Autodesk Fusion 360 part; units mm, degrees
note: some values were not read from the file. Set by a fixed rule: which sketch regions a step uses.
(part 2 of 2)
sketch "スケッチ7" plane through (0, 0, 8) normal (0, 0, 1) x (-1, 0, 0)
  arc A0 (19.6617, -4.7917) -> (19.8821, -5.409) centre (20.2564, -4.9274) ccw
  arc A1 (19.6617, -4.7917) -> (19.7936, -4.2138) centre (0, 0) ccw
  arc A2 (20.26, -3.7531) -> (19.7936, -4.2138) centre (20.3883, -4.3495) ccw
  line L0 (20.26, -3.7531) -> (20.9366, -3.6076)
  arc A3 (20.9366, -3.6076) -> (21.412, -3.0986) centre (20.8082, -3.0112) ccw
  arc A4 (21.412, -3.0986) -> (21.5646, -1.7437) centre (0, 0) ccw
  arc A5 (21.5646, -1.7437) -> (21.2144, -1.1417) centre (20.9566, -1.6945) ccw
  line L1 (21.2144, -1.1417) -> (20.5872, -0.8492)
  arc A6 (20.235, -0.2964) -> (20.5872, -0.8492) centre (20.845, -0.2964) ccw
  arc A7 (20.235, -0.2964) -> (20.235, 0.2964) centre (0, 0) ccw
  arc A8 (20.5872, 0.8492) -> (20.235, 0.2964) centre (20.845, 0.2964) ccw
  line L2 (20.5872, 0.8492) -> (21.2144, 1.1417)
  arc A9 (21.2144, 1.1417) -> (21.5646, 1.7437) centre (20.9566, 1.6945) ccw
  arc A10 (21.5646, 1.7437) -> (21.412, 3.0986) centre (0, 0) ccw
  arc A11 (21.412, 3.0986) -> (20.9366, 3.6076) centre (20.8082, 3.0112) ccw
  line L3 (20.9366, 3.6076) -> (20.26, 3.7531)
  arc A12 (19.7936, 4.2138) -> (20.26, 3.7531) centre (20.3883, 4.3495) ccw
  arc A13 (19.7936, 4.2138) -> (19.6617, 4.7917) centre (0, 0) ccw
  arc A14 (19.8821, 5.409) -> (19.6617, 4.7917) centre (20.2564, 4.9274) ccw
  line L4 (19.8821, 5.409) -> (20.4285, 5.8337)
  arc A15 (20.4285, 5.8337) -> (20.6359, 6.4986) centre (20.0541, 6.3153) ccw
  arc A16 (20.6359, 6.4986) -> (20.1856, 7.7855) centre (0, 0) ccw
  arc A17 (20.1856, 7.7855) -> (19.6089, 8.1759) centre (19.6165, 7.566) ccw
  line L5 (19.6089, 8.1759) -> (18.9169, 8.1673)
  arc A18 (18.3597, 8.5126) -> (18.9169, 8.1673) centre (18.9093, 8.7773) ccw
  arc A19 (18.3597, 8.5126) -> (18.1025, 9.0467) centre (0, 0) ccw
  arc A20 (18.18, 9.6976) -> (18.1025, 9.0467) centre (18.6521, 9.3113) ccw
  line L6 (18.18, 9.6976) -> (18.6181, 10.2332)
  arc A21 (18.6181, 10.2332) -> (18.6725, 10.9276) centre (18.146, 10.6195) ccw
  arc A22 (18.6725, 10.9276) -> (17.9471, 12.082) centre (0, 0) ccw
  arc A23 (17.9471, 12.082) -> (17.2979, 12.3343) centre (17.4411, 11.7414) ccw
  line L7 (17.2979, 12.3343) -> (16.6252, 12.172)
  arc A24 (16.0052, 12.3846) -> (16.6252, 12.172) centre (16.4821, 12.7649) ccw
  arc A25 (16.0052, 12.3846) -> (15.6356, 12.848) centre (0, 0) ccw
  arc A26 (15.5662, 13.4999) -> (15.6356, 12.848) centre (16.1125, 13.2284) ccw
  line L8 (15.5662, 13.4999) -> (15.8742, 14.1196)
  arc A27 (15.8742, 14.1196) -> (15.7727, 14.8086) centre (15.328, 14.3911) ccw
  arc A28 (15.7727, 14.8086) -> (14.8086, 15.7727) centre (0, 0) ccw
  arc A29 (14.8086, 15.7727) -> (14.1196, 15.8742) centre (14.3911, 15.328) ccw
  line L9 (14.1196, 15.8742) -> (13.4999, 15.5662)
  arc A30 (12.848, 15.6356) -> (13.4999, 15.5662) centre (13.2284, 16.1125) ccw
  arc A31 (12.848, 15.6356) -> (12.3846, 16.0052) centre (0, 0) ccw
  arc A32 (12.172, 16.6252) -> (12.3846, 16.0052) centre (12.7649, 16.4821) ccw
  line L10 (12.172, 16.6252) -> (12.3343, 17.2979)
  arc A33 (12.3343, 17.2979) -> (12.082, 17.9471) centre (11.7414, 17.4411) ccw
  arc A34 (12.082, 17.9471) -> (10.9276, 18.6725) centre (0, 0) ccw
  arc A35 (10.9276, 18.6725) -> (10.2332, 18.6181) centre (10.6195, 18.146) ccw
  line L11 (10.2332, 18.6181) -> (9.6976, 18.18)
  arc A36 (9.0467, 18.1025) -> (9.6976, 18.18) centre (9.3113, 18.6521) ccw
  arc A37 (9.0467, 18.1025) -> (8.5126, 18.3597) centre (0, 0) ccw
  arc A38 (8.1673, 18.9169) -> (8.5126, 18.3597) centre (8.7773, 18.9093) ccw
  line L12 (8.1673, 18.9169) -> (8.1759, 19.6089)
  arc A39 (8.1759, 19.6089) -> (7.7855, 20.1856) centre (7.566, 19.6165) ccw
  arc A40 (7.7855, 20.1856) -> (6.4986, 20.6359) centre (0, 0) ccw
  arc A41 (6.4986, 20.6359) -> (5.8337, 20.4285) centre (6.3153, 20.0541) ccw
  line L13 (5.8337, 20.4285) -> (5.409, 19.8821)
  arc A42 (4.7917, 19.6617) -> (5.409, 19.8821) centre (4.9274, 20.2564) ccw
  arc A43 (4.7917, 19.6617) -> (4.2138, 19.7936) centre (0, 0) ccw
  arc A44 (3.7531, 20.26) -> (4.2138, 19.7936) centre (4.3495, 20.3883) ccw
  line L14 (3.7531, 20.26) -> (3.6076, 20.9366)
  arc A45 (3.6076, 20.9366) -> (3.0986, 21.412) centre (3.0112, 20.8082) ccw
  arc A46 (3.0986, 21.412) -> (1.7437, 21.5646) centre (0, 0) ccw
  arc A47 (1.7437, 21.5646) -> (1.1417, 21.2144) centre (1.6945, 20.9566) ccw
  line L15 (1.1417, 21.2144) -> (0.8492, 20.5872)
  arc A48 (0.2964, 20.235) -> (0.8492, 20.5872) centre (0.2964, 20.845) ccw
  arc A49 (0.2964, 20.235) -> (-0.2964, 20.235) centre (0, 0) ccw
  arc A50 (-0.8492, 20.5872) -> (-0.2964, 20.235) centre (-0.2964, 20.845) ccw
  line L16 (-0.8492, 20.5872) -> (-1.1417, 21.2144)
  arc A51 (-1.1417, 21.2144) -> (-1.7437, 21.5646) centre (-1.6945, 20.9566) ccw
  arc A52 (-1.7437, 21.5646) -> (-3.0986, 21.412) centre (0, 0) ccw
  arc A53 (-3.0986, 21.412) -> (-3.6076, 20.9366) centre (-3.0112, 20.8082) ccw
  line L17 (-3.6076, 20.9366) -> (-3.7531, 20.26)
  arc A54 (-4.2138, 19.7936) -> (-3.7531, 20.26) centre (-4.3495, 20.3883) ccw
  arc A55 (-4.2138, 19.7936) -> (-4.7917, 19.6617) centre (0, 0) ccw
  arc A56 (-5.409, 19.8821) -> (-4.7917, 19.6617) centre (-4.9274, 20.2564) ccw
  line L18 (-5.409, 19.8821) -> (-5.8337, 20.4285)
  arc A57 (-5.8337, 20.4285) -> (-6.4986, 20.6359) centre (-6.3153, 20.0541) ccw
  arc A58 (-6.4986, 20.6359) -> (-7.7855, 20.1856) centre (0, 0) ccw
  arc A59 (-7.7855, 20.1856) -> (-8.1759, 19.6089) centre (-7.566, 19.6165) ccw
  line L19 (-8.1759, 19.6089) -> (-8.1673, 18.9169)
  arc A60 (-8.5126, 18.3597) -> (-8.1673, 18.9169) centre (-8.7773, 18.9093) ccw
  arc A61 (-8.5126, 18.3597) -> (-9.0467, 18.1025) centre (0, 0) ccw
  arc A62 (-9.6976, 18.18) -> (-9.0467, 18.1025) centre (-9.3113, 18.6521) ccw
  line L20 (-9.6976, 18.18) -> (-10.2332, 18.6181)
  arc A63 (-10.2332, 18.6181) -> (-10.9276, 18.6725) centre (-10.6195, 18.146) ccw
  arc A64 (-10.9276, 18.6725) -> (-12.082, 17.9471) centre (0, 0) ccw
  arc A65 (-12.082, 17.9471) -> (-12.3343, 17.2979) centre (-11.7414, 17.4411) ccw
  line L21 (-12.3343, 17.2979) -> (-12.172, 16.6252)
  arc A66 (-12.3846, 16.0052) -> (-12.172, 16.6252) centre (-12.7649, 16.4821) ccw
  arc A67 (-12.3846, 16.0052) -> (-12.848, 15.6356) centre (0, 0) ccw
  arc A68 (-13.4999, 15.5662) -> (-12.848, 15.6356) centre (-13.2284, 16.1125) ccw
  line L22 (-13.4999, 15.5662) -> (-14.1196, 15.8742)
  arc A69 (-14.1196, 15.8742) -> (-14.8086, 15.7727) centre (-14.3911, 15.328) ccw
  arc A70 (-14.8086, 15.7727) -> (-15.7727, 14.8086) centre (0, 0) ccw
  arc A71 (-15.7727, 14.8086) -> (-15.8742, 14.1196) centre (-15.328, 14.3911) ccw
  line L23 (-15.8742, 14.1196) -> (-15.5662, 13.4999)
  arc A72 (-15.6356, 12.848) -> (-15.5662, 13.4999) centre (-16.1125, 13.2284) ccw
  arc A73 (-15.6356, 12.848) -> (-16.0052, 12.3846) centre (0, 0) ccw
  arc A74 (-16.6252, 12.172) -> (-16.0052, 12.3846) centre (-16.4821, 12.7649) ccw
  line L24 (-16.6252, 12.172) -> (-17.2979, 12.3343)
  arc A75 (-17.2979, 12.3343) -> (-17.9471, 12.082) centre (-17.4411, 11.7414) ccw
  arc A76 (-17.9471, 12.082) -> (-18.6725, 10.9276) centre (0, 0) ccw
  arc A77 (-18.6725, 10.9276) -> (-18.6181, 10.2332) centre (-18.146, 10.6195) ccw
  line L25 (-18.6181, 10.2332) -> (-18.18, 9.6976)
  arc A78 (-18.1025, 9.0467) -> (-18.18, 9.6976) centre (-18.6521, 9.3113) ccw
  arc A79 (-18.1025, 9.0467) -> (-18.3597, 8.5126) centre (0, 0) ccw
  arc A80 (-18.9169, 8.1673) -> (-18.3597, 8.5126) centre (-18.9093, 8.7773) ccw
  line L26 (-18.9169, 8.1673) -> (-19.6089, 8.1759)
  arc A81 (-19.6089, 8.1759) -> (-20.1856, 7.7855) centre (-19.6165, 7.566) ccw
  arc A82 (-20.1856, 7.7855) -> (-20.6359, 6.4986) centre (0, 0) ccw
  arc A83 (-20.6359, 6.4986) -> (-20.4285, 5.8337) centre (-20.0541, 6.3153) ccw
  line L27 (-20.4285, 5.8337) -> (-19.8821, 5.409)
  arc A84 (-19.6617, 4.7917) -> (-19.8821, 5.409) centre (-20.2564, 4.9274) ccw
  arc A85 (-19.6617, 4.7917) -> (-19.7936, 4.2138) centre (0, 0) ccw
  arc A86 (-20.26, 3.7531) -> (-19.7936, 4.2138) centre (-20.3883, 4.3495) ccw
  line L28 (-20.26, 3.7531) -> (-20.9366, 3.6076)
  arc A87 (-20.9366, 3.6076) -> (-21.412, 3.0986) centre (-20.8082, 3.0112) ccw
  arc A88 (-21.412, 3.0986) -> (-21.5646, 1.7437) centre (0, 0) ccw
  arc A89 (-21.5646, 1.7437) -> (-21.2144, 1.1417) centre (-20.9566, 1.6945) ccw
  line L29 (-21.2144, 1.1417) -> (-20.5872, 0.8492)
  arc A90 (-20.235, 0.2964) -> (-20.5872, 0.8492) centre (-20.845, 0.2964) ccw
  arc A91 (-20.235, 0.2964) -> (-20.235, -0.2964) centre (0, 0) ccw
  arc A92 (-20.5872, -0.8492) -> (-20.235, -0.2964) centre (-20.845, -0.2964) ccw
  line L30 (-20.5872, -0.8492) -> (-21.2144, -1.1417)
  arc A93 (-21.2144, -1.1417) -> (-21.5646, -1.7437) centre (-20.9566, -1.6945) ccw
  arc A94 (-21.5646, -1.7437) -> (-21.412, -3.0986) centre (0, 0) ccw
  arc A95 (-21.412, -3.0986) -> (-20.9366, -3.6076) centre (-20.8082, -3.0112) ccw
  line L31 (-20.9366, -3.6076) -> (-20.26, -3.7531)
  arc A96 (-19.7936, -4.2138) -> (-20.26, -3.7531) centre (-20.3883, -4.3495) ccw
  arc A97 (-19.7936, -4.2138) -> (-19.6617, -4.7917) centre (0, 0) ccw
  arc A98 (-19.8821, -5.409) -> (-19.6617, -4.7917) centre (-20.2564, -4.9274) ccw
  line L32 (-19.8821, -5.409) -> (-20.4285, -5.8337)
  arc A99 (-20.4285, -5.8337) -> (-20.6359, -6.4986) centre (-20.0541, -6.3153) ccw
  arc A100 (-20.6359, -6.4986) -> (-20.1856, -7.7855) centre (0, 0) ccw
  arc A101 (-20.1856, -7.7855) -> (-19.6089, -8.1759) centre (-19.6165, -7.566) ccw
  line L33 (-19.6089, -8.1759) -> (-18.9169, -8.1673)
  arc A102 (-18.3597, -8.5126) -> (-18.9169, -8.1673) centre (-18.9093, -8.7773) ccw
  arc A103 (-18.3597, -8.5126) -> (-18.1025, -9.0467) centre (0, 0) ccw
  arc A104 (-18.18, -9.6976) -> (-18.1025, -9.0467) centre (-18.6521, -9.3113) ccw
  line L34 (-18.18, -9.6976) -> (-18.6181, -10.2332)
  arc A105 (-18.6181, -10.2332) -> (-18.6725, -10.9276) centre (-18.146, -10.6195) ccw
  arc A106 (-18.6725, -10.9276) -> (-17.9471, -12.082) centre (0, 0) ccw
  arc A107 (-17.9471, -12.082) -> (-17.2979, -12.3343) centre (-17.4411, -11.7414) ccw
  line L35 (-17.2979, -12.3343) -> (-16.6252, -12.172)
  arc A108 (-16.0052, -12.3846) -> (-16.6252, -12.172) centre (-16.4821, -12.7649) ccw
  arc A109 (-16.0052, -12.3846) -> (-15.6356, -12.848) centre (0, 0) ccw
  arc A110 (-15.5662, -13.4999) -> (-15.6356, -12.848) centre (-16.1125, -13.2284) ccw
  line L36 (-15.5662, -13.4999) -> (-15.8742, -14.1196)
  arc A111 (-15.8742, -14.1196) -> (-15.7727, -14.8086) centre (-15.328, -14.3911) ccw
  arc A112 (-15.7727, -14.8086) -> (-14.8086, -15.7727) centre (0, 0) ccw
  arc A113 (-14.8086, -15.7727) -> (-14.1196, -15.8742) centre (-14.3911, -15.328) ccw
  line L37 (-14.1196, -15.8742) -> (-13.4999, -15.5662)
  arc A114 (-12.848, -15.6356) -> (-13.4999, -15.5662) centre (-13.2284, -16.1125) ccw
  arc A115 (-12.848, -15.6356) -> (-12.3846, -16.0052) centre (0, 0) ccw
  arc A116 (-12.172, -16.6252) -> (-12.3846, -16.0052) centre (-12.7649, -16.4821) ccw
  line L38 (-12.172, -16.6252) -> (-12.3343, -17.2979)
  arc A117 (-12.3343, -17.2979) -> (-12.082, -17.9471) centre (-11.7414, -17.4411) ccw
  arc A118 (-12.082, -17.9471) -> (-10.9276, -18.6725) centre (0, 0) ccw
  arc A119 (-10.9276, -18.6725) -> (-10.2332, -18.6181) centre (-10.6195, -18.146) ccw
  line L39 (-10.2332, -18.6181) -> (-9.6976, -18.18)
  arc A120 (-9.0467, -18.1025) -> (-9.6976, -18.18) centre (-9.3113, -18.6521) ccw
  arc A121 (-9.0467, -18.1025) -> (-8.5126, -18.3597) centre (0, 0) ccw
  arc A122 (-8.1673, -18.9169) -> (-8.5126, -18.3597) centre (-8.7773, -18.9093) ccw
  line L40 (-8.1673, -18.9169) -> (-8.1759, -19.6089)
  arc A123 (-8.1759, -19.6089) -> (-7.7855, -20.1856) centre (-7.566, -19.6165) ccw
  arc A124 (-7.7855, -20.1856) -> (-6.4986, -20.6359) centre (0, 0) ccw
  arc A125 (-6.4986, -20.6359) -> (-5.8337, -20.4285) centre (-6.3153, -20.0541) ccw
  line L41 (-5.8337, -20.4285) -> (-5.409, -19.8821)
  arc A126 (-4.7917, -19.6617) -> (-5.409, -19.8821) centre (-4.9274, -20.2564) ccw
  arc A127 (-4.7917, -19.6617) -> (-4.2138, -19.7936) centre (0, 0) ccw
  arc A128 (-3.7531, -20.26) -> (-4.2138, -19.7936) centre (-4.3495, -20.3883) ccw
  line L42 (-3.7531, -20.26) -> (-3.6076, -20.9366)
  arc A129 (-3.6076, -20.9366) -> (-3.0986, -21.412) centre (-3.0112, -20.8082) ccw
  arc A130 (-3.0986, -21.412) -> (-1.7437, -21.5646) centre (0, 0) ccw
  arc A131 (-1.7437, -21.5646) -> (-1.1417, -21.2144) centre (-1.6945, -20.9566) ccw
  line L43 (-1.1417, -21.2144) -> (-0.8492, -20.5872)
  arc A132 (-0.2964, -20.235) -> (-0.8492, -20.5872) centre (-0.2964, -20.845) ccw
  arc A133 (-0.2964, -20.235) -> (0.2964, -20.235) centre (0, 0) ccw
  arc A134 (0.8492, -20.5872) -> (0.2964, -20.235) centre (0.2964, -20.845) ccw
  line L44 (0.8492, -20.5872) -> (1.1417, -21.2144)
  arc A135 (1.1417, -21.2144) -> (1.7437, -21.5646) centre (1.6945, -20.9566) ccw
  arc A136 (1.7437, -21.5646) -> (3.0986, -21.412) centre (0, 0) ccw
  arc A137 (3.0986, -21.412) -> (3.6076, -20.9366) centre (3.0112, -20.8082) ccw
  line L45 (3.6076, -20.9366) -> (3.7531, -20.26)
  arc A138 (4.2138, -19.7936) -> (3.7531, -20.26) centre (4.3495, -20.3883) ccw
  arc A139 (4.2138, -19.7936) -> (4.7917, -19.6617) centre (0, 0) ccw
  arc A140 (5.409, -19.8821) -> (4.7917, -19.6617) centre (4.9274, -20.2564) ccw
  line L46 (5.409, -19.8821) -> (5.8337, -20.4285)
  arc A141 (5.8337, -20.4285) -> (6.4986, -20.6359) centre (6.3153, -20.0541) ccw
  arc A142 (6.4986, -20.6359) -> (7.7855, -20.1856) centre (0, 0) ccw
  arc A143 (7.7855, -20.1856) -> (8.1759, -19.6089) centre (7.566, -19.6165) ccw
  line L47 (8.1759, -19.6089) -> (8.1673, -18.9169)
  arc A144 (8.5126, -18.3597) -> (8.1673, -18.9169) centre (8.7773, -18.9093) ccw
  arc A145 (8.5126, -18.3597) -> (9.0467, -18.1025) centre (0, 0) ccw
  arc A146 (9.6976, -18.18) -> (9.0467, -18.1025) centre (9.3113, -18.6521) ccw
  line L48 (9.6976, -18.18) -> (10.2332, -18.6181)
  arc A147 (10.2332, -18.6181) -> (10.9276, -18.6725) centre (10.6195, -18.146) ccw
  arc A148 (10.9276, -18.6725) -> (12.082, -17.9471) centre (0, 0) ccw
  arc A149 (12.082, -17.9471) -> (12.3343, -17.2979) centre (11.7414, -17.4411) ccw
  line L49 (12.3343, -17.2979) -> (12.172, -16.6252)
  arc A150 (12.3846, -16.0052) -> (12.172, -16.6252) centre (12.7649, -16.4821) ccw
  arc A151 (12.3846, -16.0052) -> (12.848, -15.6356) centre (0, 0) ccw
  arc A152 (13.4999, -15.5662) -> (12.848, -15.6356) centre (13.2284, -16.1125) ccw
  line L50 (13.4999, -15.5662) -> (14.1196, -15.8742)
  arc A153 (14.1196, -15.8742) -> (14.8086, -15.7727) centre (14.3911, -15.328) ccw
  arc A154 (14.8086, -15.7727) -> (15.7727, -14.8086) centre (0, 0) ccw
  arc A155 (15.7727, -14.8086) -> (15.8742, -14.1196) centre (15.328, -14.3911) ccw
  line L51 (15.8742, -14.1196) -> (15.5662, -13.4999)
  arc A156 (15.6356, -12.848) -> (15.5662, -13.4999) centre (16.1125, -13.2284) ccw
  arc A157 (15.6356, -12.848) -> (16.0052, -12.3846) centre (0, 0) ccw
  arc A158 (16.6252, -12.172) -> (16.0052, -12.3846) centre (16.4821, -12.7649) ccw
  line L52 (16.6252, -12.172) -> (17.2979, -12.3343)
  arc A159 (17.2979, -12.3343) -> (17.9471, -12.082) centre (17.4411, -11.7414) ccw
  arc A160 (17.9471, -12.082) -> (18.6725, -10.9276) centre (0, 0) ccw
  arc A161 (18.6725, -10.9276) -> (18.6181, -10.2332) centre (18.146, -10.6195) ccw
  line L53 (18.6181, -10.2332) -> (18.18, -9.6976)
  arc A162 (18.1025, -9.0467) -> (18.18, -9.6976) centre (18.6521, -9.3113) ccw
  arc A163 (18.1025, -9.0467) -> (18.3597, -8.5126) centre (0, 0) ccw
  arc A164 (18.9169, -8.1673) -> (18.3597, -8.5126) centre (18.9093, -8.7773) ccw
  line L54 (18.9169, -8.1673) -> (19.6089, -8.1759)
  arc A165 (19.6089, -8.1759) -> (20.1856, -7.7855) centre (19.6165, -7.566) ccw
  arc A166 (20.1856, -7.7855) -> (20.6359, -6.4986) centre (0, 0) ccw
  arc A167 (20.6359, -6.4986) -> (20.4285, -5.8337) centre (20.0541, -6.3153) ccw
  line L55 (20.4285, -5.8337) -> (19.8821, -5.409)
  line L56 (-0.3, 3) -> (0.3, 3)
  line L57 (0.3, 3) -> (0.3, -3)
  line L58 (0.3, -3) -> (-0.3, -3)
  line L59 (-0.3, -3) -> (-0.3, 3)
  line L60 (-0.3, 3) -> (0.3, -3) construction
  line L61 (0.3, 3) -> (-0.3, -3) construction
  circle A168 centre (-0.3, 0) radius 3
  circle A169 centre (0.3, 0) radius 3
  dimension "d78" = 0.6
  dimension "d79" = 6
  constraint horizontal L56
  constraint perpendicular L56 L57
  constraint parallel L56 L58
  constraint parallel L57 L59
  constraint coincident L60 A1.centre
  constraint coincident L61 A1.centre
  constraint coincident A1.centre A4.centre
  constraint midpoint L59 A168.centre
  constraint coincident L58.end A168
  constraint midpoint L57 A169.centre
  constraint coincident L57.end A169
  measures "d78" distance of L57.end L58.end
  measures "d79" distance of L56.end L57.end
extrude "押し出し7" cut sketch "スケッチ7" against normal blind 8 contours L59 A168 A169 | L57 A168 A169 | L59 A169 | L57 A168 picked at (-2.9825, -0.8024) picked at (3.04, 0.5606)
cylinder "円柱プリミティブ1" cut diameter 8 height -8 placed x (1, 0, 0) y (0, 1, 0) z (0, 0, 1) at (0, 0, 8)
sketch "スケッチ9" plane through (0, 0, 8) normal (0, 0, 1) x (-1, 0, 0)
  circle A0 centre (0, 0) radius 4
  arc A1 (19.6617, -4.7917) -> (19.8821, -5.409) centre (20.2564, -4.9274) ccw
  arc A2 (19.6617, -4.7917) -> (19.7936, -4.2138) centre (0, 0) ccw
  arc A3 (20.26, -3.7531) -> (19.7936, -4.2138) centre (20.3883, -4.3495) ccw
  line L0 (20.26, -3.7531) -> (20.9366, -3.6076)
  arc A4 (20.9366, -3.6076) -> (21.412, -3.0986) centre (20.8082, -3.0112) ccw
  arc A5 (21.412, -3.0986) -> (21.5646, -1.7437) centre (0, 0) ccw
  arc A6 (21.5646, -1.7437) -> (21.2144, -1.1417) centre (20.9566, -1.6945) ccw
  line L1 (21.2144, -1.1417) -> (20.5872, -0.8492)
  arc A7 (20.235, -0.2964) -> (20.5872, -0.8492) centre (20.845, -0.2964) ccw
  arc A8 (20.235, -0.2964) -> (20.235, 0.2964) centre (0, 0) ccw
  arc A9 (20.5872, 0.8492) -> (20.235, 0.2964) centre (20.845, 0.2964) ccw
  line L2 (20.5872, 0.8492) -> (21.2144, 1.1417)
  arc A10 (21.2144, 1.1417) -> (21.5646, 1.7437) centre (20.9566, 1.6945) ccw
  arc A11 (21.5646, 1.7437) -> (21.412, 3.0986) centre (0, 0) ccw
  arc A12 (21.412, 3.0986) -> (20.9366, 3.6076) centre (20.8082, 3.0112) ccw
  line L3 (20.9366, 3.6076) -> (20.26, 3.7531)
  arc A13 (19.7936, 4.2138) -> (20.26, 3.7531) centre (20.3883, 4.3495) ccw
  arc A14 (19.7936, 4.2138) -> (19.6617, 4.7917) centre (0, 0) ccw
  arc A15 (19.8821, 5.409) -> (19.6617, 4.7917) centre (20.2564, 4.9274) ccw
  line L4 (19.8821, 5.409) -> (20.4285, 5.8337)
  arc A16 (20.4285, 5.8337) -> (20.6359, 6.4986) centre (20.0541, 6.3153) ccw
  arc A17 (20.6359, 6.4986) -> (20.1856, 7.7855) centre (0, 0) ccw
  arc A18 (20.1856, 7.7855) -> (19.6089, 8.1759) centre (19.6165, 7.566) ccw
  line L5 (19.6089, 8.1759) -> (18.9169, 8.1673)
  arc A19 (18.3597, 8.5126) -> (18.9169, 8.1673) centre (18.9093, 8.7773) ccw
  arc A20 (18.3597, 8.5126) -> (18.1025, 9.0467) centre (0, 0) ccw
  arc A21 (18.18, 9.6976) -> (18.1025, 9.0467) centre (18.6521, 9.3113) ccw
  line L6 (18.18, 9.6976) -> (18.6181, 10.2332)
  arc A22 (18.6181, 10.2332) -> (18.6725, 10.9276) centre (18.146, 10.6195) ccw
  arc A23 (18.6725, 10.9276) -> (17.9471, 12.082) centre (0, 0) ccw
  arc A24 (17.9471, 12.082) -> (17.2979, 12.3343) centre (17.4411, 11.7414) ccw
  line L7 (17.2979, 12.3343) -> (16.6252, 12.172)
  arc A25 (16.0052, 12.3846) -> (16.6252, 12.172) centre (16.4821, 12.7649) ccw
  arc A26 (16.0052, 12.3846) -> (15.6356, 12.848) centre (0, 0) ccw
  arc A27 (15.5662, 13.4999) -> (15.6356, 12.848) centre (16.1125, 13.2284) ccw
  line L8 (15.5662, 13.4999) -> (15.8742, 14.1196)
  arc A28 (15.8742, 14.1196) -> (15.7727, 14.8086) centre (15.328, 14.3911) ccw
  arc A29 (15.7727, 14.8086) -> (14.8086, 15.7727) centre (0, 0) ccw
  arc A30 (14.8086, 15.7727) -> (14.1196, 15.8742) centre (14.3911, 15.328) ccw
  line L9 (14.1196, 15.8742) -> (13.4999, 15.5662)
  arc A31 (12.848, 15.6356) -> (13.4999, 15.5662) centre (13.2284, 16.1125) ccw
  arc A32 (12.848, 15.6356) -> (12.3846, 16.0052) centre (0, 0) ccw
  arc A33 (12.172, 16.6252) -> (12.3846, 16.0052) centre (12.7649, 16.4821) ccw
  line L10 (12.172, 16.6252) -> (12.3343, 17.2979)
  arc A34 (12.3343, 17.2979) -> (12.082, 17.9471) centre (11.7414, 17.4411) ccw
  arc A35 (12.082, 17.9471) -> (10.9276, 18.6725) centre (0, 0) ccw
  arc A36 (10.9276, 18.6725) -> (10.2332, 18.6181) centre (10.6195, 18.146) ccw
  line L11 (10.2332, 18.6181) -> (9.6976, 18.18)
  arc A37 (9.0467, 18.1025) -> (9.6976, 18.18) centre (9.3113, 18.6521) ccw
  arc A38 (9.0467, 18.1025) -> (8.5126, 18.3597) centre (0, 0) ccw
  arc A39 (8.1673, 18.9169) -> (8.5126, 18.3597) centre (8.7773, 18.9093) ccw
  line L12 (8.1673, 18.9169) -> (8.1759, 19.6089)
  arc A40 (8.1759, 19.6089) -> (7.7855, 20.1856) centre (7.566, 19.6165) ccw
  arc A41 (7.7855, 20.1856) -> (6.4986, 20.6359) centre (0, 0) ccw
  arc A42 (6.4986, 20.6359) -> (5.8337, 20.4285) centre (6.3153, 20.0541) ccw
  line L13 (5.8337, 20.4285) -> (5.409, 19.8821)
  arc A43 (4.7917, 19.6617) -> (5.409, 19.8821) centre (4.9274, 20.2564) ccw
  arc A44 (4.7917, 19.6617) -> (4.2138, 19.7936) centre (0, 0) ccw
  arc A45 (3.7531, 20.26) -> (4.2138, 19.7936) centre (4.3495, 20.3883) ccw
  line L14 (3.7531, 20.26) -> (3.6076, 20.9366)
  arc A46 (3.6076, 20.9366) -> (3.0986, 21.412) centre (3.0112, 20.8082) ccw
  arc A47 (3.0986, 21.412) -> (1.7437, 21.5646) centre (0, 0) ccw
  arc A48 (1.7437, 21.5646) -> (1.1417, 21.2144) centre (1.6945, 20.9566) ccw
  line L15 (1.1417, 21.2144) -> (0.8492, 20.5872)
  arc A49 (0.2964, 20.235) -> (0.8492, 20.5872) centre (0.2964, 20.845) ccw
  arc A50 (0.2964, 20.235) -> (-0.2964, 20.235) centre (0, 0) ccw
  arc A51 (-0.8492, 20.5872) -> (-0.2964, 20.235) centre (-0.2964, 20.845) ccw
  line L16 (-0.8492, 20.5872) -> (-1.1417, 21.2144)
  arc A52 (-1.1417, 21.2144) -> (-1.7437, 21.5646) centre (-1.6945, 20.9566) ccw
  arc A53 (-1.7437, 21.5646) -> (-3.0986, 21.412) centre (0, 0) ccw
  arc A54 (-3.0986, 21.412) -> (-3.6076, 20.9366) centre (-3.0112, 20.8082) ccw
  line L17 (-3.6076, 20.9366) -> (-3.7531, 20.26)
  arc A55 (-4.2138, 19.7936) -> (-3.7531, 20.26) centre (-4.3495, 20.3883) ccw
  arc A56 (-4.2138, 19.7936) -> (-4.7917, 19.6617) centre (0, 0) ccw
  arc A57 (-5.409, 19.8821) -> (-4.7917, 19.6617) centre (-4.9274, 20.2564) ccw
  line L18 (-5.409, 19.8821) -> (-5.8337, 20.4285)
  arc A58 (-5.8337, 20.4285) -> (-6.4986, 20.6359) centre (-6.3153, 20.0541) ccw
  arc A59 (-6.4986, 20.6359) -> (-7.7855, 20.1856) centre (0, 0) ccw
  arc A60 (-7.7855, 20.1856) -> (-8.1759, 19.6089) centre (-7.566, 19.6165) ccw
  line L19 (-8.1759, 19.6089) -> (-8.1673, 18.9169)
  arc A61 (-8.5126, 18.3597) -> (-8.1673, 18.9169) centre (-8.7773, 18.9093) ccw
  arc A62 (-8.5126, 18.3597) -> (-9.0467, 18.1025) centre (0, 0) ccw
  arc A63 (-9.6976, 18.18) -> (-9.0467, 18.1025) centre (-9.3113, 18.6521) ccw
  line L20 (-9.6976, 18.18) -> (-10.2332, 18.6181)
  arc A64 (-10.2332, 18.6181) -> (-10.9276, 18.6725) centre (-10.6195, 18.146) ccw
  arc A65 (-10.9276, 18.6725) -> (-12.082, 17.9471) centre (0, 0) ccw
  arc A66 (-12.082, 17.9471) -> (-12.3343, 17.2979) centre (-11.7414, 17.4411) ccw
  line L21 (-12.3343, 17.2979) -> (-12.172, 16.6252)
  arc A67 (-12.3846, 16.0052) -> (-12.172, 16.6252) centre (-12.7649, 16.4821) ccw
  arc A68 (-12.3846, 16.0052) -> (-12.848, 15.6356) centre (0, 0) ccw
  arc A69 (-13.4999, 15.5662) -> (-12.848, 15.6356) centre (-13.2284, 16.1125) ccw
  line L22 (-13.4999, 15.5662) -> (-14.1196, 15.8742)
  arc A70 (-14.1196, 15.8742) -> (-14.8086, 15.7727) centre (-14.3911, 15.328) ccw
  arc A71 (-14.8086, 15.7727) -> (-15.7727, 14.8086) centre (0, 0) ccw
  arc A72 (-15.7727, 14.8086) -> (-15.8742, 14.1196) centre (-15.328, 14.3911) ccw
  line L23 (-15.8742, 14.1196) -> (-15.5662, 13.4999)
  arc A73 (-15.6356, 12.848) -> (-15.5662, 13.4999) centre (-16.1125, 13.2284) ccw
  arc A74 (-15.6356, 12.848) -> (-16.0052, 12.3846) centre (0, 0) ccw
  arc A75 (-16.6252, 12.172) -> (-16.0052, 12.3846) centre (-16.4821, 12.7649) ccw
  line L24 (-16.6252, 12.172) -> (-17.2979, 12.3343)
  arc A76 (-17.2979, 12.3343) -> (-17.9471, 12.082) centre (-17.4411, 11.7414) ccw
  arc A77 (-17.9471, 12.082) -> (-18.6725, 10.9276) centre (0, 0) ccw
  arc A78 (-18.6725, 10.9276) -> (-18.6181, 10.2332) centre (-18.146, 10.6195) ccw
  line L25 (-18.6181, 10.2332) -> (-18.18, 9.6976)
  arc A79 (-18.1025, 9.0467) -> (-18.18, 9.6976) centre (-18.6521, 9.3113) ccw
  arc A80 (-18.1025, 9.0467) -> (-18.3597, 8.5126) centre (0, 0) ccw
  arc A81 (-18.9169, 8.1673) -> (-18.3597, 8.5126) centre (-18.9093, 8.7773) ccw
  line L26 (-18.9169, 8.1673) -> (-19.6089, 8.1759)
  arc A82 (-19.6089, 8.1759) -> (-20.1856, 7.7855) centre (-19.6165, 7.566) ccw
  arc A83 (-20.1856, 7.7855) -> (-20.6359, 6.4986) centre (0, 0) ccw
  arc A84 (-20.6359, 6.4986) -> (-20.4285, 5.8337) centre (-20.0541, 6.3153) ccw
  line L27 (-20.4285, 5.8337) -> (-19.8821, 5.409)
  arc A85 (-19.6617, 4.7917) -> (-19.8821, 5.409) centre (-20.2564, 4.9274) ccw
  arc A86 (-19.6617, 4.7917) -> (-19.7936, 4.2138) centre (0, 0) ccw
  arc A87 (-20.26, 3.7531) -> (-19.7936, 4.2138) centre (-20.3883, 4.3495) ccw
  line L28 (-20.26, 3.7531) -> (-20.9366, 3.6076)
  arc A88 (-20.9366, 3.6076) -> (-21.412, 3.0986) centre (-20.8082, 3.0112) ccw
  arc A89 (-21.412, 3.0986) -> (-21.5646, 1.7437) centre (0, 0) ccw
  arc A90 (-21.5646, 1.7437) -> (-21.2144, 1.1417) centre (-20.9566, 1.6945) ccw
  line L29 (-21.2144, 1.1417) -> (-20.5872, 0.8492)
  arc A91 (-20.235, 0.2964) -> (-20.5872, 0.8492) centre (-20.845, 0.2964) ccw
  arc A92 (-20.235, 0.2964) -> (-20.235, -0.2964) centre (0, 0) ccw
  arc A93 (-20.5872, -0.8492) -> (-20.235, -0.2964) centre (-20.845, -0.2964) ccw
  line L30 (-20.5872, -0.8492) -> (-21.2144, -1.1417)
  arc A94 (-21.2144, -1.1417) -> (-21.5646, -1.7437) centre (-20.9566, -1.6945) ccw
  arc A95 (-21.5646, -1.7437) -> (-21.412, -3.0986) centre (0, 0) ccw
  arc A96 (-21.412, -3.0986) -> (-20.9366, -3.6076) centre (-20.8082, -3.0112) ccw
  line L31 (-20.9366, -3.6076) -> (-20.26, -3.7531)
  arc A97 (-19.7936, -4.2138) -> (-20.26, -3.7531) centre (-20.3883, -4.3495) ccw
  arc A98 (-19.7936, -4.2138) -> (-19.6617, -4.7917) centre (0, 0) ccw
  arc A99 (-19.8821, -5.409) -> (-19.6617, -4.7917) centre (-20.2564, -4.9274) ccw
  line L32 (-19.8821, -5.409) -> (-20.4285, -5.8337)
  arc A100 (-20.4285, -5.8337) -> (-20.6359, -6.4986) centre (-20.0541, -6.3153) ccw
  arc A101 (-20.6359, -6.4986) -> (-20.1856, -7.7855) centre (0, 0) ccw
  arc A102 (-20.1856, -7.7855) -> (-19.6089, -8.1759) centre (-19.6165, -7.566) ccw
  line L33 (-19.6089, -8.1759) -> (-18.9169, -8.1673)
  arc A103 (-18.3597, -8.5126) -> (-18.9169, -8.1673) centre (-18.9093, -8.7773) ccw
  arc A104 (-18.3597, -8.5126) -> (-18.1025, -9.0467) centre (0, 0) ccw
  arc A105 (-18.18, -9.6976) -> (-18.1025, -9.0467) centre (-18.6521, -9.3113) ccw
  line L34 (-18.18, -9.6976) -> (-18.6181, -10.2332)
  arc A106 (-18.6181, -10.2332) -> (-18.6725, -10.9276) centre (-18.146, -10.6195) ccw
  arc A107 (-18.6725, -10.9276) -> (-17.9471, -12.082) centre (0, 0) ccw
  arc A108 (-17.9471, -12.082) -> (-17.2979, -12.3343) centre (-17.4411, -11.7414) ccw
  line L35 (-17.2979, -12.3343) -> (-16.6252, -12.172)
  arc A109 (-16.0052, -12.3846) -> (-16.6252, -12.172) centre (-16.4821, -12.7649) ccw
  arc A110 (-16.0052, -12.3846) -> (-15.6356, -12.848) centre (0, 0) ccw
  arc A111 (-15.5662, -13.4999) -> (-15.6356, -12.848) centre (-16.1125, -13.2284) ccw
  line L36 (-15.5662, -13.4999) -> (-15.8742, -14.1196)
  arc A112 (-15.8742, -14.1196) -> (-15.7727, -14.8086) centre (-15.328, -14.3911) ccw
  arc A113 (-15.7727, -14.8086) -> (-14.8086, -15.7727) centre (0, 0) ccw
  arc A114 (-14.8086, -15.7727) -> (-14.1196, -15.8742) centre (-14.3911, -15.328) ccw
  line L37 (-14.1196, -15.8742) -> (-13.4999, -15.5662)
  arc A115 (-12.848, -15.6356) -> (-13.4999, -15.5662) centre (-13.2284, -16.1125) ccw
  arc A116 (-12.848, -15.6356) -> (-12.3846, -16.0052) centre (0, 0) ccw
  arc A117 (-12.172, -16.6252) -> (-12.3846, -16.0052) centre (-12.7649, -16.4821) ccw
  line L38 (-12.172, -16.6252) -> (-12.3343, -17.2979)
  arc A118 (-12.3343, -17.2979) -> (-12.082, -17.9471) centre (-11.7414, -17.4411) ccw
  arc A119 (-12.082, -17.9471) -> (-10.9276, -18.6725) centre (0, 0) ccw
  arc A120 (-10.9276, -18.6725) -> (-10.2332, -18.6181) centre (-10.6195, -18.146) ccw
  line L39 (-10.2332, -18.6181) -> (-9.6976, -18.18)
  arc A121 (-9.0467, -18.1025) -> (-9.6976, -18.18) centre (-9.3113, -18.6521) ccw
  arc A122 (-9.0467, -18.1025) -> (-8.5126, -18.3597) centre (0, 0) ccw
  arc A123 (-8.1673, -18.9169) -> (-8.5126, -18.3597) centre (-8.7773, -18.9093) ccw
  line L40 (-8.1673, -18.9169) -> (-8.1759, -19.6089)
  arc A124 (-8.1759, -19.6089) -> (-7.7855, -20.1856) centre (-7.566, -19.6165) ccw
  arc A125 (-7.7855, -20.1856) -> (-6.4986, -20.6359) centre (0, 0) ccw
  arc A126 (-6.4986, -20.6359) -> (-5.8337, -20.4285) centre (-6.3153, -20.0541) ccw
  line L41 (-5.8337, -20.4285) -> (-5.409, -19.8821)
  arc A127 (-4.7917, -19.6617) -> (-5.409, -19.8821) centre (-4.9274, -20.2564) ccw
  arc A128 (-4.7917, -19.6617) -> (-4.2138, -19.7936) centre (0, 0) ccw
  arc A129 (-3.7531, -20.26) -> (-4.2138, -19.7936) centre (-4.3495, -20.3883) ccw
  line L42 (-3.7531, -20.26) -> (-3.6076, -20.9366)
  arc A130 (-3.6076, -20.9366) -> (-3.0986, -21.412) centre (-3.0112, -20.8082) ccw
  arc A131 (-3.0986, -21.412) -> (-1.7437, -21.5646) centre (0, 0) ccw
  arc A132 (-1.7437, -21.5646) -> (-1.1417, -21.2144) centre (-1.6945, -20.9566) ccw
  line L43 (-1.1417, -21.2144) -> (-0.8492, -20.5872)
  arc A133 (-0.2964, -20.235) -> (-0.8492, -20.5872) centre (-0.2964, -20.845) ccw
  arc A134 (-0.2964, -20.235) -> (0.2964, -20.235) centre (0, 0) ccw
  arc A135 (0.8492, -20.5872) -> (0.2964, -20.235) centre (0.2964, -20.845) ccw
  line L44 (0.8492, -20.5872) -> (1.1417, -21.2144)
  arc A136 (1.1417, -21.2144) -> (1.7437, -21.5646) centre (1.6945, -20.9566) ccw
  arc A137 (1.7437, -21.5646) -> (3.0986, -21.412) centre (0, 0) ccw
  arc A138 (3.0986, -21.412) -> (3.6076, -20.9366) centre (3.0112, -20.8082) ccw
  line L45 (3.6076, -20.9366) -> (3.7531, -20.26)
  arc A139 (4.2138, -19.7936) -> (3.7531, -20.26) centre (4.3495, -20.3883) ccw
  arc A140 (4.2138, -19.7936) -> (4.7917, -19.6617) centre (0, 0) ccw
  arc A141 (5.409, -19.8821) -> (4.7917, -19.6617) centre (4.9274, -20.2564) ccw
  line L46 (5.409, -19.8821) -> (5.8337, -20.4285)
  arc A142 (5.8337, -20.4285) -> (6.4986, -20.6359) centre (6.3153, -20.0541) ccw
  arc A143 (6.4986, -20.6359) -> (7.7855, -20.1856) centre (0, 0) ccw
  arc A144 (7.7855, -20.1856) -> (8.1759, -19.6089) centre (7.566, -19.6165) ccw
  line L47 (8.1759, -19.6089) -> (8.1673, -18.9169)
  arc A145 (8.5126, -18.3597) -> (8.1673, -18.9169) centre (8.7773, -18.9093) ccw
  arc A146 (8.5126, -18.3597) -> (9.0467, -18.1025) centre (0, 0) ccw
  arc A147 (9.6976, -18.18) -> (9.0467, -18.1025) centre (9.3113, -18.6521) ccw
  line L48 (9.6976, -18.18) -> (10.2332, -18.6181)
  arc A148 (10.2332, -18.6181) -> (10.9276, -18.6725) centre (10.6195, -18.146) ccw
  arc A149 (10.9276, -18.6725) -> (12.082, -17.9471) centre (0, 0) ccw
  arc A150 (12.082, -17.9471) -> (12.3343, -17.2979) centre (11.7414, -17.4411) ccw
  line L49 (12.3343, -17.2979) -> (12.172, -16.6252)
  arc A151 (12.3846, -16.0052) -> (12.172, -16.6252) centre (12.7649, -16.4821) ccw
  arc A152 (12.3846, -16.0052) -> (12.848, -15.6356) centre (0, 0) ccw
  arc A153 (13.4999, -15.5662) -> (12.848, -15.6356) centre (13.2284, -16.1125) ccw
  line L50 (13.4999, -15.5662) -> (14.1196, -15.8742)
  arc A154 (14.1196, -15.8742) -> (14.8086, -15.7727) centre (14.3911, -15.328) ccw
  arc A155 (14.8086, -15.7727) -> (15.7727, -14.8086) centre (0, 0) ccw
  arc A156 (15.7727, -14.8086) -> (15.8742, -14.1196) centre (15.328, -14.3911) ccw
  line L51 (15.8742, -14.1196) -> (15.5662, -13.4999)
  arc A157 (15.6356, -12.848) -> (15.5662, -13.4999) centre (16.1125, -13.2284) ccw
  arc A158 (15.6356, -12.848) -> (16.0052, -12.3846) centre (0, 0) ccw
  arc A159 (16.6252, -12.172) -> (16.0052, -12.3846) centre (16.4821, -12.7649) ccw
  line L52 (16.6252, -12.172) -> (17.2979, -12.3343)
  arc A160 (17.2979, -12.3343) -> (17.9471, -12.082) centre (17.4411, -11.7414) ccw
  arc A161 (17.9471, -12.082) -> (18.6725, -10.9276) centre (0, 0) ccw
  arc A162 (18.6725, -10.9276) -> (18.6181, -10.2332) centre (18.146, -10.6195) ccw
  line L53 (18.6181, -10.2332) -> (18.18, -9.6976)
  arc A163 (18.1025, -9.0467) -> (18.18, -9.6976) centre (18.6521, -9.3113) ccw
  arc A164 (18.1025, -9.0467) -> (18.3597, -8.5126) centre (0, 0) ccw
  arc A165 (18.9169, -8.1673) -> (18.3597, -8.5126) centre (18.9093, -8.7773) ccw
  line L54 (18.9169, -8.1673) -> (19.6089, -8.1759)
  arc A166 (19.6089, -8.1759) -> (20.1856, -7.7855) centre (19.6165, -7.566) ccw
  arc A167 (20.1856, -7.7855) -> (20.6359, -6.4986) centre (0, 0) ccw
  arc A168 (20.6359, -6.4986) -> (20.4285, -5.8337) centre (20.0541, -6.3153) ccw
  line L55 (20.4285, -5.8337) -> (19.8821, -5.409)
  circle A169 centre (0, 0) radius 10
  line L56 (0, 0) -> (-10, 0)
  circle A170 centre (-10, 0) radius 1.7
  circle A171 centre (0, -10) radius 1.7
  circle A172 centre (10, 0) radius 1.7
  circle A173 centre (0, 10) radius 1.7
  dimension "d84" = 20
  dimension "d85" = 3.4
  dimension "d87" = 360
  constraint coincident A0.centre A2.centre
  constraint coincident A169 L56.end
  constraint horizontal L56
  constraint coincident L56.end A170.centre
  measures "d84" diameter of A169
  measures "d85" diameter of A170
extrude "押し出し8" cut sketch "スケッチ9" against normal blind 8 contours A169 A172 | A169 A172 | A169 A173 | A169 A173 | A169 A171 | A169 A171 | A169 L56 A170 | A169 A170 | A169 L56 A170
